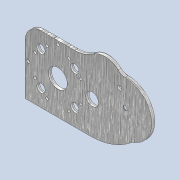
# Autodesk Inventor part: 中間フレーム
Saved by Autodesk Inventor 2020.4 (Build 244396000, 396)
## iProperties
Created: 2021-04-23
Part Number: 中間フレーム
Material: アルミニウム 7075
Document SubType Name: Modeling
Designer: happy
Density: 2.81 g/cm^3
Appearance: サテン - ブラシ仕上げ 重厚
Mass: 54.3319 g
Surface Area: 148.325 cm^2
Volume: 19.3352 cm^3
Author: happy
Autodesk Inventor part; units mm, degrees
ref_plane "YZ Plane" through (0, 0, 0) normal (1, 0, 0) x (0, 1, 0)
ref_plane "XZ Plane" through (0, 0, 0) normal (0, 1, 0) x (-1, 0, 0)
ref_plane "XY Plane" through (0, 0, 0) normal (0, 0, 1) x (1, 0, 0)
sketch "スケッチ1" plane through (0, 0, 0) normal (0, 0, 1) x (1, 0, 0)
  line L0 (65.0196, -14.5) -> (65.0196, 33.6804)
  circle A0 centre (80.0196, 33.6804) radius 15 construction
  line L1 (80.0196, 48.6804) -> (112.2, 48.6804)
  circle A1 centre (112.2, 33.6804) radius 15 construction
  line L2 (127.2, -14.5) -> (65.0196, -14.5)
  circle A2 centre (80.0196, 33.6804) radius 3.05 construction
  circle A3 centre (112.2, 33.6804) radius 3.05 construction
  circle A4 centre (112.2, 1.5) radius 3.05 construction
  circle A5 centre (80.0196, 1.5) radius 3.05 construction
  circle A6 centre (96.1098, 17.5902) radius 2.85 construction
  circle A7 centre (128.7687, 16.8502) radius 5.7 construction
  circle A8 centre (160, 25) radius 21.5 construction
  circle A9 centre (128.7687, 16.8502) radius 28.5 construction
  circle A10 centre (128.7687, 16.8502) radius 29.4672 construction
  circle A11 centre (160, 25) radius 25.8772 construction
  circle A12 centre (80.0196, 33.6804) radius 4
  circle A13 centre (112.2, 33.6804) radius 4
  circle A14 centre (80.0196, 1.5) radius 4
  circle A15 centre (112.2, 1.5) radius 4
  arc A16 (112.2, 48.6804) -> (130.0806, 54.5913) centre (112.2, 78.6804) ccw
  arc A17 (153.3164, 53.0826) -> (160, 50.3812) centre (160, 60) ccw
  arc A18 (153.3164, 53.0826) -> (130.0806, 54.5913) centre (140.809, 40.1379) ccw
  circle A19 centre (96.1098, 17.5902) radius 9.025
  circle A20 centre (128.7687, 16.8502) radius 6.025
  circle A21 centre (160, 25) radius 2
  arc A22 (168.6809, 1.1495) -> (160, 50.3812) centre (160, 25) ccw
  arc A23 (168.6809, 1.1495) -> (165.807, -0.5048) centre (171.9707, -7.8892) ccw
  circle A24 centre (171.9707, -7.8892) radius 8.6188 construction
  arc A25 (127.2, -14.5) -> (165.807, -0.5048) centre (127.2, 45.748) ccw
  circle A26 centre (160, 60) radius 8.6188 construction
  circle A27 centre (154.8697, 39.0954) radius 3 construction
  circle A28 centre (154.8697, 39.0954) radius 2
  arc A29 (158.348, 26.1273) -> (99.1742, 26.079) centre (128.7687, 16.8502) ccw construction
  arc A30 (98.7866, 8.9713) -> (159.1095, 23.2092) centre (128.7687, 16.8502) ccw construction
  arc A31 (80.0196, 48.6804) -> (65.0196, 33.6804) centre (80.0196, 33.6804) ccw
  circle A32 centre (68.0196, 17.5902) radius 1.5
  circle A33 centre (96.1098, 45.6804) radius 1.5
  circle A34 centre (74.3628, 28.0235) radius 1.3
  circle A35 centre (85.6765, 39.3372) radius 1.3
  circle A36 centre (106.5431, 39.3372) radius 1.3
  circle A37 centre (117.8569, 28.0235) radius 1.3
  circle A38 centre (117.8569, 7.1569) radius 1.3
  circle A39 centre (106.5431, -4.1569) radius 1.3
  circle A40 centre (85.6765, -4.1569) radius 1.3
  circle A41 centre (74.3628, 7.1569) radius 1.3
  line L3 (74.3628, 28.0235) -> (85.6765, 39.3372) construction
  point P0 (0, 0)
  point P1 (0, 0)
  point P2 (96.1924, 17.5902)
  point P3 (80.1022, 1.5)
  point P4 (112.2826, 1.5)
  point P5 (112.2826, 33.6804)
  point P6 (80.1962, 33.857)
  point P7 (160, 60)
  dimension "d0" = 8
  dimension "d1" = 30
  dimension "d2" = 18.05
  dimension "d3" = 12.05
  dimension "d4" = 4
  dimension "d5" = 1
  dimension "d6" = 18
  dimension "d7" = 4
  dimension "d8" = 31
  dimension "d9" = 32.2772
  dimension "d10" = 60.248
  dimension "d13" = 3
  dimension "d14" = 3
  dimension "d15" = 2.6
  dimension "d16" = 16
  constraints: 40 centre point, 22 point on circle, 11 equal radius, 9 coincident, 9 tangent, 8 end point, 3 concentric, 2 horizontal, 2 vertical alignment, 1 midpoint, 1 point on line, 1 vertical, 29 other
  measures "d0" diameter of A13
  measures "d1" radius of A16
  measures "d2" diameter of A19
  measures "d3" diameter of A20
  measures "d4" diameter of A21
  measures "d5" radial gap between concentric circles of A24 A23
  measures "d6" radius of A18
  measures "d7" diameter of A28
  measures "d8" radius of A29
  measures "d9" distance of A20.centre A21.centre
  measures "d10" radius of A25
  measures "d13" diameter of A32
  measures "d14" diameter of A33
  measures "d15" diameter of A34
  measures "d16" distance of L3.end L3.start
extrude "押し出し1" add sketch "スケッチ1" along normal blind 3
chamfer "面取り1" distance 2.5 angle 45 1 edges at (158, 25, 0)
